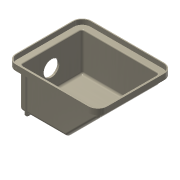
# Autodesk Inventor part: Air-Box
Saved by Autodesk Inventor 2022 Beta2 (Build 260130000, 130) ContinuousBuild 0
## iProperties
Shininess: 64.0
Length Units: 11269
Angle Units: 11279
Time Units: 11290
Mass Units: 11283
Length Display Precision: 3
Angle Display Precision: 2
Compacted: True
Part Number: Air-Box
Document SubType Name: Modeling
Created: 2004-03-26
Designer: Administrator
Manufacturer: Standard
Standards Organization: Custom
Density: 1 g/cm^3
Mass: 510.979 g
Surface Area: 3365.03 cm^2
Volume: 510.979 cm^3
Material: Generic
Appearance: Light Beige
Density: 0.0
Volumn: 0.0
Area: 0.0
PropertySet Name: Model Information
Control State: 0
Master: False
Checked Out: False
Author: Administrator
Autodesk Inventor part; units mm, degrees
ref_plane "YZ Plane" through (0, 0, 0) normal (1, 0, 0) x (0, 1, 0)
ref_plane "XZ Plane" through (0, 0, 0) normal (0, 1, 0) x (-1, 0, 0)
ref_plane "XY Plane" through (0, 0, 0) normal (0, 0, 1) x (1, 0, 0)
sketch "Sketch1" plane through (0, 0, 0) normal (0, 0, 1) x (1, 0, 0)
  line L0 (0, 0) -> (250, 0)
  line L1 (250, 0) -> (250, 200)
  line L2 (250, 200) -> (0, 200)
  line L3 (0, 200) -> (0, 0)
  dimension "d0" = 200
  dimension "d1" = 250
  constraints: 8 end point, 2 parallel, 1 horizontal, 1 perpendicular
  measures "d0" distance of L2.end L0.start
  measures "d1" distance of L1.end L2.end
extrude "Extrusion1" add sketch "Sketch1" against normal blind 25
ref_plane "Work Plane1" through (0, 100, 0) normal (0, -1, 0) x (1, 0, 0)
sketch "Sketch2" plane through (0, 100, 0) normal (0, -1, 0) x (1, 0, 0)
  line L0 (0, -25) -> (0, -125)
  line L1 (0, -125) -> (150, -125)
  line L2 (150, -125) -> (250, -25)
  line L3 (0, -25) -> (250, -25)
  dimension "d4" = 100
  dimension "d5" = 150
  dimension "d7" = 45
  constraints: 8 end point, 1 parallel, 1 perpendicular, 1 vertical
  measures "d4" distance of L0.start L0.end
  measures "d5" distance of L0.end L1.end
  measures "d7" angle of L2 L1
extrude "Extrusion2" add sketch "Sketch2" along normal mid plane 200
fillet "Fillet1" radius 10 11 edges at (0, 200, -62.5) (0, 0, -62.5) (250, 0, -12.5) (250, 200, -12.5) (200, 0, -75) (200, 200, -75) (75, 200, -125) (150, 100, -125) (75, 0, -125) (0, 100, -125) (250, 100, -25)
shell "Shell1" thickness 3 removed faces 1 at (86.6667, 133.3333, 0)
sketch "Sketch3" plane through (0, 0, 0) normal (0, 0, 1) x (1, 0, 0)
  arc A0 (0, 10) -> (10, 0) centre (10, 10) ccw projected
  line L0 (10, 0) -> (240, 0) projected
  arc A1 (240, 0) -> (250, 10) centre (240, 10) ccw projected
  line L1 (250, 10) -> (250, 190) projected
  arc A2 (250, 190) -> (240, 200) centre (240, 190) ccw projected
  line L2 (240, 200) -> (10, 200) projected
  arc A3 (10, 200) -> (0, 190) centre (10, 190) ccw projected
  line L3 (0, 190) -> (0, 10) projected
  arc A4 (-20, 10) -> (10, -20) centre (10, 10) ccw
  line L4 (10, -20) -> (240, -20)
  arc A5 (240, -20) -> (270, 10) centre (240, 10) ccw
  line L5 (270, 10) -> (270, 190)
  arc A6 (270, 190) -> (240, 220) centre (240, 190) ccw
  line L6 (240, 220) -> (10, 220)
  arc A7 (10, 220) -> (-20, 190) centre (10, 190) ccw
  line L7 (-20, 190) -> (-20, 10)
  dimension "d12" = 20
  constraints: 8 end point, 8 point on circle, 4 centre point, 7 other
  measures "d12" distance between parallel lines of L7 L3
extrude "Extrusion3" add sketch "Sketch3" against normal blind 3
sketch "Sketch4" plane through (0, 0, 0) normal (0, 0, 1) x (1, 0, 0)
  arc A0 (-20, 10) -> (10, -20) centre (10, 10) ccw projected
  line L0 (10, -20) -> (240, -20) projected
  arc A1 (240, -20) -> (270, 10) centre (240, 10) ccw projected
  line L1 (270, 10) -> (270, 190) projected
  arc A2 (270, 190) -> (240, 220) centre (240, 190) ccw projected
  line L2 (240, 220) -> (10, 220) projected
  arc A3 (10, 220) -> (-20, 190) centre (10, 190) ccw projected
  line L3 (-20, 190) -> (-20, 10) projected
  arc A4 (-17, 10) -> (10, -17) centre (10, 10) ccw
  line L4 (10, -17) -> (240, -17)
  arc A5 (240, -17) -> (267, 10) centre (240, 10) ccw
  line L5 (267, 10) -> (267, 190)
  arc A6 (267, 190) -> (240, 217) centre (240, 190) ccw
  line L6 (240, 217) -> (10, 217)
  arc A7 (10, 217) -> (-17, 190) centre (10, 190) ccw
  line L7 (-17, 190) -> (-17, 10)
  dimension "d15" = 3
  constraints: 8 end point, 8 point on circle, 4 centre point, 7 other
  measures "d15" distance between parallel lines of L3 L7
extrude "Extrusion4" add sketch "Sketch4" along normal blind 15
sketch "Sketch5" plane through (0, 10, -115) normal (-1, 0, 0) x (0, 0, 1)
  line L0 (0, 180) -> (112, 180) projected
  line L1 (0, 0) -> (0, 180) projected
  circle A0 centre (56, 90) radius 32.5
  point P0 (56, 180)
  point P1 (0, 90)
  dimension "d18" = 65
  constraints: 2 midpoint, 1 centre point, 1 horizontal alignment, 1 vertical alignment
  measures "d18" diameter of A0
extrude "Extrusion5" add sketch "Sketch5" along normal blind 3
sketch "Sketch6" plane through (-3, 100, -59) normal (-1, 0, 0) x (0, 0, 1)
  circle A0 centre (0, 0) radius 32.5 projected
hole "Hole1" at (-3, 100, -59) direction (1, 0, 0) diameter 50 depth 6 tip angle 118
fillet "Fillet2" radius 3 8 edges at (125, 3, 0) (5.0503, 5.0503, 0) (3, 100, 0) (5.0503, 194.9497, 0) (125, 197, 0) (244.9497, 194.9497, 0) (247, 100, 0) (244.9497, 5.0503, 0)
fillet "Fillet3" radius 6 8 edges at (250, 100, -3) (247.0711, 2.9289, -3) (125, 0, -3) (2.9289, 2.9289, -3) (0, 100, -3) (2.9289, 197.0711, -3) (125, 200, -3) (247.0711, 197.0711, -3)
sketch "Sketch7" plane through (-3, 100, -59) normal (-1, 0, 0) x (0, 0, 1)
  circle A0 centre (0, 0) radius 25 projected
  circle A1 centre (0, 0) radius 32.5 projected
  line L0 (0, 0) -> (42.8212, 0) construction
  point P0 (28.75, 0)
  dimension "d30" = 28.75
  constraints: 2 end point, 1 horizontal, 1 point on line
  measures "d30" distance of point (28.75, 0) A0.centre
hole "Hole2" at (-3, 100, -30.25) direction (1, 0, 0) diameter 4.134 depth 6 tip angle 118 thread size "M5x0.8" class "6H" standard "ANSI Metric M Profile"
ref_plane "Work Plane2" through (145.8579, 190, -130) normal (0, 0, -1) x (-1, 0, 0)
sketch "Sketch8" plane through (145.8579, 190, -130) normal (0, 0, -1) x (-1, 0, 0)
  line L0 (135.8579, 16) -> (-94.1421, 16) projected
  line L1 (-94.1421, -196) -> (135.8579, -196) projected
  line L2 (0, 0) -> (135.8579, 0) projected
  line L3 (135.8579, -180) -> (0, -180) projected
  line L4 (120.8579, 16) -> (120.8579, -196)
  dimension "d42" = 15
  constraints: 2 end point, 2 point on line, 1 perpendicular
  measures "d42" distance from line of L0.start L4
rib "Rib1" sketch "Sketch8" thickness 3 direction (0, 0, 1) end up to next extend profile no curves L4
fillet "Fillet4" radius 10 2 edges at (25, 206, -130) (25, -6, -130)
hole "Hole4" at (10, -20, 6) direction (0, 1, 0) diameter 3 depth 8 tip angle 118
equation "\"d8\" = d0"
equation "\"d13\" = d11"
equation "\"d15\" = d11"
equation "\"d11\" = 3"
body "Solid1"
